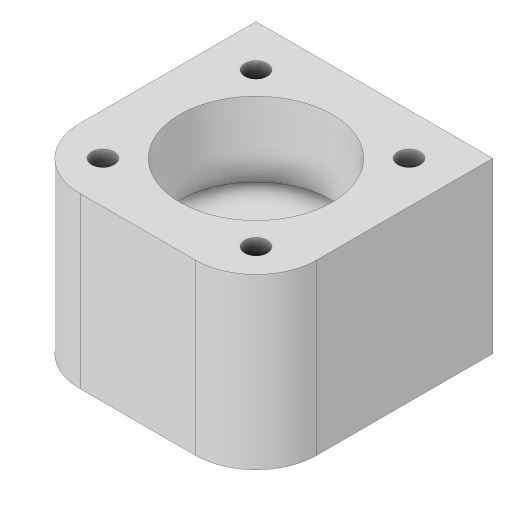
# Autodesk Inventor part: PART_!
Saved by Autodesk Inventor 2024 (Build 280153000, 153)
## iProperties
Created: 2024-08-20
Part Number: PART_!
Material: Generic
Document SubType Name: Modeling
Designer: Jhuliams
Density: 1 g/cm^3
Appearance: Default
Author: Jhuliams
Autodesk Inventor part; units mm, degrees
ref_plane "YZ Plane" through (0, 0, 0) normal (1, 0, 0) x (0, 1, 0)
ref_plane "XZ Plane" through (0, 0, 0) normal (0, 1, 0) x (-1, 0, 0)
ref_plane "XY Plane" through (0, 0, 0) normal (0, 0, 1) x (1, 0, 0)
sketch "Sketch1" plane through (0, 0, 0) normal (0, 1, 0) x (-1, 0, 0)
  line L0 (17.5, 17.5) -> (-17.5, 17.5)
  line L1 (-17.5, 17.5) -> (-17.5, -17.5)
  line L2 (-17.5, -17.5) -> (17.5, -17.5)
  line L3 (17.5, -17.5) -> (17.5, 17.5)
  line L4 (17.5, 17.5) -> (-17.5, -17.5) construction
  line L5 (-17.5, 17.5) -> (17.5, -17.5) construction
  point P0 (0, 0)
  dimension "d0" = 35
  dimension "d1" = 35
  constraints: 12 end point, 2 midpoint, 2 parallel, 1 horizontal, 1 perpendicular
  measures "d0" distance of L2.end L1.end
  measures "d1" distance of L1.end L0.end
extrude "Extrusion1" add sketch "Sketch1" along normal mid plane 25
sketch "Sketch2" plane through (0, 12.5, 0) normal (0, 1, 0) x (1, 0, 0)
  circle A0 centre (0, 0) radius 4.15
  dimension "d4" = 8.3
  constraints: 1 centre point, 1 coincident
  measures "d4" diameter of A0
extrude "Extrusion2" cut sketch "Sketch2" against normal blind 25
sketch "Sketch3" plane through (0, 12.5, 0) normal (0, 1, 0) x (1, 0, 0)
  circle A0 centre (0, 0) radius 11.25
  dimension "d7" = 22.5
  constraints: 1 centre point, 1 coincident
  measures "d7" diameter of A0
extrude "Extrusion3" cut sketch "Sketch3" against normal blind 11
sketch "Sketch4" plane through (0, 12.5, 0) normal (0, 1, 0) x (1, 0, 0)
  circle A0 centre (0, 0) radius 4.15 projected
  circle A1 centre (0, 0) radius 16
  line L0 (17.5, 17.5) -> (-17.5, 17.5) projected
  line L1 (-17.5, -17.5) -> (17.5, -17.5) projected
  line L2 (17.5, 17.5) -> (-17.5, -17.5)
  line L3 (-17.5, 17.5) -> (17.5, -17.5)
  circle A2 centre (11.3137, 11.3137) radius 1.65
  circle A3 centre (-11.3137, 11.3137) radius 1.65
  circle A4 centre (-11.3137, -11.3137) radius 1.65
  circle A5 centre (11.3137, -11.3137) radius 1.65
  dimension "d10" = 32
  dimension "d11" = 3.3
  dimension "d14" = 360
  constraints: 4 centre point, 4 end point, 1 coincident, 1 point on line, 12 other
  measures "d11" diameter of A2
extrude "Extrusion4" cut sketch "Sketch4" against normal blind 25 contours A2 A1 L2 | L2 A1 A2 | A5 A1 L3 | L3 A1 A5 | A3 A1 L3 | L3 A1 A3 | L2 A2 A1 | A1 A2 L2 | A4 A1 L2 | L2 A1 A4 | L3 A5 A1 | A1 A5 L3 | L3 A3 A1 | A1 A3 L3 | L2 A4 A1 | A1 A4 L2
fillet "Fillet1" radius 9 2 edges at (-17.5, 0, -17.5) (-17.5, 0, 17.5)
mirror "Mirror1" about plane through (0, 0, 0) normal (0, 1, 0) of "Extrusion3"
body "Solid1"
